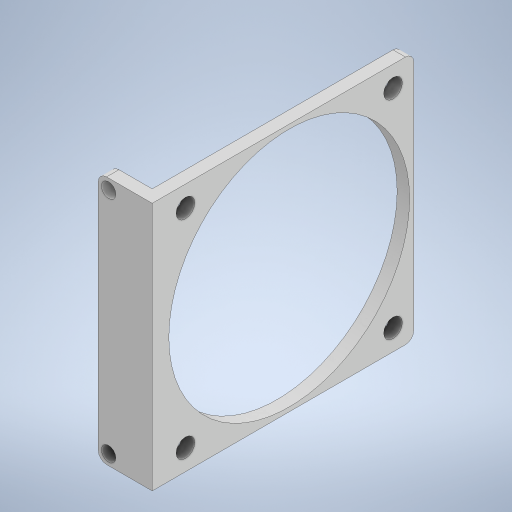
# Autodesk Inventor part: Halter_Lüfter
Saved by Autodesk Inventor 2024 (Build 280153000, 153)
## iProperties
Created: 2024-11-28
Part Number: Halter_Lüfter
Material: Generisch
Document SubType Name: Modeling
Designer: month
Density: 1 g/cm^3
Appearance: Vorgabe
Author: month
Autodesk Inventor part; units mm, degrees
ref_plane "YZ Plane" through (0, 0, 0) normal (1, 0, 0) x (0, 1, 0)
ref_plane "XZ Plane" through (0, 0, 0) normal (0, 1, 0) x (-1, 0, 0)
ref_plane "XY Plane" through (0, 0, 0) normal (0, 0, 1) x (1, 0, 0)
sketch "Skizze1" plane through (0, 0, 0) normal (1, 0, 0) x (0, 1, 0)
  line L0 (0, 0) -> (60, 0)
  line L1 (60, 0) -> (60, -60)
  line L2 (60, -60) -> (0, -60)
  line L3 (0, -60) -> (0, 0)
  line L4 (0, -30) -> (60, -30) construction
  line L5 (30, 0) -> (30, -60) construction
  circle A0 centre (30, -30) radius 29
  line L6 (0, -5) -> (60, -5) construction
  line L7 (60, -55) -> (0, -55) construction
  line L8 (5, 0) -> (5, -60) construction
  line L9 (55, -60) -> (55, 0) construction
  circle A1 centre (55, -5) radius 2.25
  circle A2 centre (55, -55) radius 2.25
  circle A3 centre (5, -55) radius 2.25
  circle A4 centre (5, -5) radius 2.25
  dimension "d0" = 60
  dimension "d1" = 60
  dimension "d2" = 58
  dimension "d3" = 5
  dimension "d4" = 5
  dimension "d5" = 5
  dimension "d6" = 5
  dimension "d7" = 4.5
  dimension "d8" = 4.5
  dimension "d9" = 4.5
  dimension "d10" = 4.5
  constraints: 20 end point, 16 point on line, 5 centre point, 5 midpoint, 5 perpendicular, 2 parallel, 1 horizontal
  measures "d0" distance of L2.end L0.start
  measures "d1" distance of L1.end L2.end
  measures "d2" diameter of A0
  measures "d3" distance between parallel lines of L0 L6
  measures "d4" distance between parallel lines of L2 L7
  measures "d5" distance between parallel lines of L1 L9
  measures "d6" distance between parallel lines of L3 L8
  measures "d7" diameter of A1
  measures "d8" diameter of A2
  measures "d9" diameter of A4
  measures "d10" diameter of A3
extrude "Extrusion1" add sketch "Skizze1" against normal blind 3
sketch "Skizze2" plane through (0, 0, -60) normal (0, -1, 0) x (1, 0, 0)
  line L0 (0, 60) -> (-13, 60)
  line L1 (-13, 60) -> (-13, 0)
  line L2 (-13, 0) -> (0, 0)
  line L3 (-1.5, 60) -> (-1.5, 0) construction
  line L4 (0, 60) -> (-3, 60) projected
  line L5 (0, 60) -> (0, 0) projected
  line L6 (-10.5, 0) -> (-10.5, 60) construction
  line L7 (5, 57.5) -> (-13, 57.5) construction
  line L8 (5, 2.5) -> (-13, 2.5) construction
  circle A0 centre (-10.5, 57.5) radius 1.75
  circle A1 centre (-10.5, 2.5) radius 1.75
  line L9 (0, 60) -> (0, 0)
  point P0 (-3, 0)
  dimension "d13" = 13
  dimension "d14" = 1.5
  dimension "d17" = 2.5
  dimension "d18" = 2.5
  dimension "d19" = 2.5
  dimension "d21" = 3.5
  dimension "d23" = 3.5
  constraints: 16 end point, 14 point on line, 5 perpendicular, 2 centre point, 1 horizontal, 1 parallel, 1 symmetric about line, 1 vertical
  measures "d13" distance of L0.start L0.end
  measures "d14" distance between parallel lines of L3 L5
  measures "d17" distance between parallel lines of L1 L6
  measures "d18" distance between parallel lines of L0 L7
  measures "d19" distance between parallel lines of L2 L8
  measures "d21" diameter of A0
  measures "d23" diameter of A1
fillet "Rundung1" radius 2 2 edges at (-1.5, 60, -60) (-1.5, 60, 0)
extrude "Extrusion4" add sketch "Skizze2" along normal blind 3
fillet "Rundung2" radius 2 2 edges at (-13, -1.5, 0) (-13, -1.5, -60)
